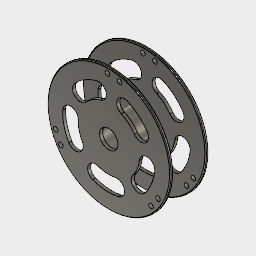
80x40 Spool v3 (Autodesk Fusion 360 design; units mm, degrees)
Autodesk Fusion 360 part; units mm, degrees
note: some values were not read from the file. Set by a fixed rule: which sketch regions a step uses.
sketch "Sketch1" plane through (0, 0, 0) normal (0, 1, 0) x (1, 0, 0)
  circle A0 centre (0, 0) radius 40
  dimension "d5" = 80
  measures "d5" diameter of A0
extrude "Extrude1" add sketch "Sketch1" along normal blind 2 makes body 1
sketch "Sketch2" plane through (0, 0, 0) normal (0, 1, 0) x (1, 0, 0)
  circle A0 centre (0, 0) radius 6
  dimension "d10" = 12
  measures "d10" diameter of A0
sketch "Sketch3" plane through (0, 0, 0) normal (0, -1, 0) x (1, 0, 0)
  circle A0 centre (0, 0) radius 40
  circle A1 centre (0, 0) radius 7
  dimension "d13" = 14
  measures "d13" diameter of A1
extrude "Extrude3" add sketch "Sketch3" along normal blind 5 contours A1 bodies 1
sketch "Sketch4" plane through (0, 0, 0) normal (0, -1, 0) x (1, 0, 0)
  circle A0 centre (0, 0) radius 7
  circle A1 centre (0, 0) radius 40
  circle A2 centre (0, 0) radius 8.5
  dimension "d16" = 17
  measures "d16" diameter of A2
extrude "Extrude4" add sketch "Sketch4" along normal blind 21 separate body contours A2 makes body 2
sketch "Sketch5" plane through (0, -21, 0) normal (0, -1, 0) x (1, 0, 0)
  circle A0 centre (0, 0) radius 7
  circle A1 centre (0, 0) radius 8.5
  circle A2 centre (0, 0) radius 40
  circle A3 centre (0, 0) radius 6
  dimension "d19" = 80
  dimension "d20" = 12
  measures "d19" diameter of A2
  measures "d20" diameter of A3
extrude "Extrude5" add sketch "Sketch5" along normal blind 2 contours A0 | A1 | A2 | A3 bodies 2
sketch "Sketch6" plane through (0, 2, 0) normal (0, 1, 0) x (-1, 0, 0)
  circle A0 centre (0, 0) radius 40
  circle A1 centre (0, 0) radius 6
  dimension "d23" = 12
  measures "d23" diameter of A1
extrude "Extrude6" cut sketch "Sketch6" against normal blind 25 contours A1 bodies 1 2
fillet "Fillet1" radius 0.5 4 edges at (-37.2931, 0, 14.4646) (-37.2931, 2, 14.4646) (-37.2931, -23, -14.4646) (-37.2931, -21, -14.4646) on bodies 1 2
sketch "Sketch8" plane through (0, -23, 0) normal (0, -1, 0) x (1, 0, 0)
  circle A0 centre (0, 0) radius 6
  circle A1 centre (0, 0) radius 39.5
  circle A2 centre (0, 0) radius 12.5 construction
  arc A3 (-5.3359, 19.2751) -> (-14.8615, 13.3841) centre (0, 0) ccw
  arc A4 (-5.3359, 19.2751) -> (-8.0039, 28.9126) centre (-6.6699, 24.0938) ccw
  arc A5 (-8.0039, 28.9126) -> (-22.2923, 20.0762) centre (0, 0) ccw
  arc A6 (-22.2923, 20.0762) -> (-14.8615, 13.3841) centre (-18.5769, 16.7301) ccw
  arc A7 (-6.6699, 24.0938) -> (-18.5769, 16.7301) centre (0, 0) ccw construction
  dimension "d40" = 25
  dimension "d48" = 14
  dimension "d50" = 5
  dimension "d61" = 25
  measures "d40" diameter of A2
  measures "d48" distance of A6.centre A4.centre
  measures "d50" radius of A4
  measures "d61" radius of A7
extrude "Extrude11" cut sketch "Sketch8" against normal blind 25 contours A3 A4 A5 A6 bodies 1 2
pattern_circular "C-Pattern2" count 5 over 360 about axis through (0, -23, 0) along (0, -1, 0) of "Extrude11"
sketch "Sketch9" plane through (0, -23, 0) normal (0, -1, 0) x (1, 0, 0)
  circle A0 centre (0, 0) radius 6
  circle A1 centre (-0.8375, 36.4904) radius 1.5
  circle A2 centre (0, 0) radius 39.5
  arc A3 (16.6828, 11.0311) -> (8.1366, 18.2701) centre (0, 0) ccw
  arc A4 (12.2049, 27.4051) -> (8.1366, 18.2701) centre (10.1707, 22.8376) ccw
  arc A5 (25.0241, 16.5467) -> (12.2049, 27.4051) centre (0, 0) ccw
  arc A6 (16.6828, 11.0311) -> (25.0241, 16.5467) centre (20.8535, 13.7889) ccw
  arc A7 (15.6465, -12.4575) -> (19.8902, -2.0926) centre (0, 0) ccw
  arc A8 (29.8353, -3.1389) -> (19.8902, -2.0926) centre (24.8628, -2.6157) ccw
  arc A9 (23.4697, -18.6862) -> (29.8353, -3.1389) centre (0, 0) ccw
  arc A10 (15.6465, -12.4575) -> (23.4697, -18.6862) centre (19.5581, -15.5718) ccw
  arc A11 (-7.0127, -18.7302) -> (4.1563, -19.5634) centre (0, 0) ccw
  arc A12 (6.2344, -29.3451) -> (4.1563, -19.5634) centre (5.1953, -24.4542) ccw
  arc A13 (-10.5191, -28.0954) -> (6.2344, -29.3451) centre (0, 0) ccw
  arc A14 (-7.0127, -18.7302) -> (-10.5191, -28.0954) centre (-8.7659, -23.4128) ccw
  arc A15 (-19.9806, 0.8815) -> (-17.3215, -9.9982) centre (0, 0) ccw
  arc A16 (-25.9823, -14.9974) -> (-17.3215, -9.9982) centre (-21.6519, -12.4978) ccw
  arc A17 (-29.9708, 1.3223) -> (-25.9823, -14.9974) centre (0, 0) ccw
  arc A18 (-19.9806, 0.8815) -> (-29.9708, 1.3223) centre (-24.9757, 1.1019) ccw
  arc A19 (-8.0039, 28.9126) -> (-22.2923, 20.0762) centre (0, 0) ccw
  arc A20 (-5.3359, 19.2751) -> (-8.0039, 28.9126) centre (-6.6699, 24.0938) ccw
  arc A21 (-5.3359, 19.2751) -> (-14.8615, 13.3841) centre (0, 0) ccw
  arc A22 (-22.2923, 20.0762) -> (-14.8615, 13.3841) centre (-18.5769, 16.7301) ccw
  circle A23 centre (0, 0) radius 36.5
  line L0 (0, 0) -> (7.0277, 35.8171)
  circle A24 centre (7.0277, 35.8171) radius 1.5
  dimension "d55" = 3
  dimension "d65" = 3
  dimension "d67" = 73
  measures "d55" diameter of A1
  measures "d65" diameter of A24
  measures "d67" diameter of A23
extrude "Extrude12" cut sketch "Sketch9" against normal blind 25 contours A1 A23 | A1 A23 | A23 A24 | A23 L0 A24 | A23 L0 A24 bodies 1 2
pattern_circular "C-Pattern4" count 3 over 360 about axis through (0, -23, 0) along (0, 1, 0) of "Extrude12"
equation "RimDIAM = 80 mm"
equation "spokeDIAOUT = 14 mm"
equation "AxelDIA = 12 mm"
equation "outerspokeDIA = spokeDIAOUT + spokethinkness"
equation "d5 = RimDIAM"
equation "RimTHICK = 2 mm"
equation "CenterSpace = OverallThickness - ( RimTHICK * 2 )"
equation "d8 = RimTHICK"
equation "d10 = AxelDIA"
equation "d13 = spokeDIAOUT"
equation "d16 = outerspokeDIA"
equation "d17 = CenterSpace"
equation "d19 = RimDIAM"
equation "d20 = AxelDIA"
equation "d21 = RimTHICK"
equation "d23 = AxelDIA"
equation "OverallThickness = 25 mm"
equation "d25 = -OverallThickness"
equation "RimHolePattencentreline = 25 mm"
equation "RimHoleRAID = 5 mm"
equation "d40 = RimHolePattencentreline"
equation "Numberofholes = 5"
equation "spokethinkness = 3 mm"
equation "d48 = rimholelength"
equation "rimholelength = 14 mm"
equation "d50 = RimHoleRAID"
equation "d51 = -OverallThickness"
equation "d53 = Numberofholes"
equation "d57 = -OverallThickness"
equation "d61 = RimHolePattencentreline"
equation "Cableendholes = RimDIAM - 7 mm"
equation "d67 = Cableendholes"
